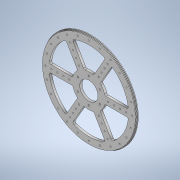
# Autodesk Inventor part: IndexerWheelV2
Saved by Autodesk Inventor 2020 (Build 240168000, 168)
## iProperties
Created: 2020-01-26
Part Number: IndexerWheelV2
Material: Generic
Document SubType Name: Modeling
Designer: srini
Density: 1 g/cm^3
Appearance: Default
Author: srini
Autodesk Inventor part; units mm, degrees
ref_plane "YZ Plane" through (0, 0, 0) normal (1, 0, 0) x (0, 1, 0)
ref_plane "XZ Plane" through (0, 0, 0) normal (0, 1, 0) x (-1, 0, 0)
ref_plane "XY Plane" through (0, 0, 0) normal (0, 0, 1) x (1, 0, 0)
sketch "Sketch1" plane through (0, 0, 0) normal (0, 0, 1) x (1, 0, 0)
  circle A0 centre (0, 0) radius 200.025
  circle A1 centre (0, 0) radius 38.4
  circle A2 centre (0, 53.975) radius 3.3734
  circle A3 centre (-46.7437, 26.9875) radius 3.3734
  circle A4 centre (-46.7437, -26.9875) radius 3.3734
  circle A5 centre (0, -53.975) radius 3.3734
  circle A6 centre (46.7437, -26.9875) radius 3.3734
  circle A7 centre (46.7437, 26.9875) radius 3.3734
  arc A8 (70.0141, 153.018) -> (-70.0141, 153.018) centre (0, 0) ccw
  line L0 (-70.0141, 153.018) -> (-20.2629, 66.8464)
  arc A9 (20.2629, 66.8464) -> (-20.2629, 66.8464) centre (0, 0) ccw
  line L1 (20.2629, 66.8464) -> (70.0141, 153.018)
  line L2 (0, 168.275) -> (0, 69.85) construction
  arc A10 (-97.5104, 137.143) -> (-167.5245, 15.875) centre (0, 0) ccw
  line L3 (-167.5245, 15.875) -> (-68.0221, 15.875)
  arc A11 (-47.7592, 50.9714) -> (-68.0221, 15.875) centre (0, 0) ccw
  line L4 (-47.7592, 50.9714) -> (-97.5104, 137.143)
  arc A12 (-167.5245, -15.875) -> (-97.5104, -137.143) centre (0, 0) ccw
  line L5 (-97.5104, -137.143) -> (-47.7592, -50.9714)
  arc A13 (-68.0221, -15.875) -> (-47.7592, -50.9714) centre (0, 0) ccw
  line L6 (-68.0221, -15.875) -> (-167.5245, -15.875)
  arc A14 (-70.0141, -153.018) -> (70.0141, -153.018) centre (0, 0) ccw
  line L7 (70.0141, -153.018) -> (20.2629, -66.8464)
  arc A15 (-20.2629, -66.8464) -> (20.2629, -66.8464) centre (0, 0) ccw
  line L8 (-20.2629, -66.8464) -> (-70.0141, -153.018)
  arc A16 (97.5104, -137.143) -> (167.5245, -15.875) centre (0, 0) ccw
  line L9 (167.5245, -15.875) -> (68.0221, -15.875)
  arc A17 (47.7592, -50.9714) -> (68.0221, -15.875) centre (0, 0) ccw
  line L10 (47.7592, -50.9714) -> (97.5104, -137.143)
  arc A18 (167.5245, 15.875) -> (97.5104, 137.143) centre (0, 0) ccw
  line L11 (97.5104, 137.143) -> (47.7592, 50.9714)
  arc A19 (68.0221, 15.875) -> (47.7592, 50.9714) centre (0, 0) ccw
  line L12 (68.0221, 15.875) -> (167.5245, 15.875)
  point P0 (-145.7304, 84.1375)
  point P1 (-60.4919, 34.925)
  point P2 (-145.7304, -84.1375)
  point P3 (-60.4919, -34.925)
  point P4 (0, -168.275)
  point P5 (0, -69.85)
  point P6 (145.7304, -84.1375)
  point P7 (60.4919, -34.925)
  point P8 (145.7304, 84.1375)
  point P9 (60.4919, 34.925)
  dimension "d0" = 400.05
  dimension "d1" = 76.8
  dimension "d2" = 53.975
  dimension "d3" = 6.7469
  dimension "d6" = 360
  dimension "d8" = 168.275
  dimension "d9" = 69.85
  dimension "d12" = 360
  dimension "d14" = 31.75
  constraints: 26 end point, 26 point on circle, 20 centre point, 2 coincident, 2 concentric, 1 parallel, 1 point on line, 1 vertical, 1 vertical alignment, 86 other
  measures "d0" diameter of A0
  measures "d1" diameter of A1
  measures "d2" distance of point (0, 0) A2.centre
  measures "d3" diameter of A2
  measures "d8" radius of A8
  measures "d9" radius of A9
  measures "d14" distance between parallel lines of L4 L0
extrude "Extrusion1" add sketch "Sketch1" along normal blind 9.525
fillet "Fillet1" radius 6.35 24 edges at (-167.5245, 15.875, 4.7625) (-70.0141, 153.018, 4.7625) (97.5104, 137.143, 4.7625) (167.5245, -15.875, 4.7625) (70.0141, -153.018, 4.7625) (-97.5104, -137.143, 4.7625) (-167.5245, -15.875, 4.7625) (-97.5104, 137.143, 4.7625) (70.0141, 153.018, 4.7625) (167.5245, 15.875, 4.7625) (97.5104, -137.143, 4.7625) (-70.0141, -153.018, 4.7625) (-68.0221, -15.875, 4.7625) (-47.7592, -50.9714, 4.7625) (-20.2629, -66.8464, 4.7625) (20.2629, -66.8464, 4.7625) (47.7592, -50.9714, 4.7625) (68.0221, -15.875, 4.7625) (68.0221, 15.875, 4.7625) (47.7592, 50.9714, 4.7625) (20.2629, 66.8464, 4.7625) (-20.2629, 66.8464, 4.7625) (-47.7592, 50.9714, 4.7625) (-68.0221, 15.875, 4.7625)
sketch "Sketch2" plane through (0, 0, 9.525) normal (0, 0, 1) x (1, 0, 0)
  circle A0 centre (0, 0) radius 198.4375
  circle A1 centre (0, 0) radius 200.025 projected
  dimension "d18" = 1.5875
  constraints: 1 centre point, 1 coincident
  measures "d18" radial gap between concentric circles of A0 A1
extrude "Extrusion2" cut sketch "Sketch2" against normal blind 6.35
sketch "Sketch3" plane through (0, 0, 9.525) normal (0, 0, 1) x (1, 0, 0)
  circle A0 centre (0, 0) radius 196.85
  circle A1 centre (0, 0) radius 198.4375 projected
  dimension "d21" = 1.5875
  constraints: 1 centre point, 1 coincident
  measures "d21" radial gap between concentric circles of A0 A1
extrude "Extrusion3" cut sketch "Sketch3" against normal blind 3.175
sketch "Sketch5" plane through (0, 0, 9.525) normal (0, 0, 1) x (1, 0, 0)
  circle A0 centre (-184.15, 0) radius 2.5781
  line L0 (-72.8868, 15.875) -> (-160.3925, 15.875) projected
  circle A1 centre (-158.75, 0) radius 2.5781
  circle A2 centre (-133.35, 0) radius 2.5781
  circle A3 centre (-107.95, 0) radius 2.5781
  circle A4 centre (-82.55, 0) radius 2.5781
  circle A5 centre (-79.375, -137.4815) radius 2.5781
  circle A6 centre (-66.675, -115.4845) radius 2.5781
  circle A7 centre (-53.975, -93.4874) radius 2.5781
  circle A8 centre (-41.275, -71.4904) radius 2.5781
  circle A9 centre (79.375, -137.4815) radius 2.5781
  circle A10 centre (66.675, -115.4845) radius 2.5781
  circle A11 centre (53.975, -93.4874) radius 2.5781
  circle A12 centre (41.275, -71.4904) radius 2.5781
  circle A13 centre (158.75, 0) radius 2.5781
  circle A14 centre (133.35, 0) radius 2.5781
  circle A15 centre (107.95, 0) radius 2.5781
  circle A16 centre (82.55, 0) radius 2.5781
  circle A17 centre (79.375, 137.4815) radius 2.5781
  circle A18 centre (66.675, 115.4845) radius 2.5781
  circle A19 centre (53.975, 93.4874) radius 2.5781
  circle A20 centre (41.275, 71.4904) radius 2.5781
  circle A21 centre (-79.375, 137.4815) radius 2.5781
  circle A22 centre (-66.675, 115.4845) radius 2.5781
  circle A23 centre (-53.975, 93.4874) radius 2.5781
  circle A24 centre (-41.275, 71.4904) radius 2.5781
  circle A25 centre (-177.8752, 47.6615) radius 2.5781
  circle A26 centre (-159.4786, 92.075) radius 2.5781
  circle A27 centre (-130.2137, 130.2137) radius 2.5781
  circle A28 centre (-92.075, 159.4786) radius 2.5781
  circle A29 centre (-47.6615, 177.8752) radius 2.5781
  circle A30 centre (0, 184.15) radius 2.5781
  circle A31 centre (47.6615, 177.8752) radius 2.5781
  circle A32 centre (92.075, 159.4786) radius 2.5781
  circle A33 centre (130.2137, 130.2137) radius 2.5781
  circle A34 centre (159.4786, 92.075) radius 2.5781
  circle A35 centre (177.8752, 47.6615) radius 2.5781
  circle A36 centre (184.15, 0) radius 2.5781
  circle A37 centre (177.8752, -47.6615) radius 2.5781
  circle A38 centre (159.4786, -92.075) radius 2.5781
  circle A39 centre (130.2137, -130.2137) radius 2.5781
  circle A40 centre (92.075, -159.4786) radius 2.5781
  circle A41 centre (47.6615, -177.8752) radius 2.5781
  circle A42 centre (0, -184.15) radius 2.5781
  circle A43 centre (-47.6615, -177.8752) radius 2.5781
  circle A44 centre (-92.075, -159.4786) radius 2.5781
  circle A45 centre (-130.2137, -130.2137) radius 2.5781
  circle A46 centre (-159.4786, -92.075) radius 2.5781
  circle A47 centre (-177.8752, -47.6615) radius 2.5781
  point P0 (0, 0)
  dimension "d24" = 5.1562
  dimension "d25" = 184.15
  dimension "d28" = 25.4
  dimension "d35" = 360
  dimension "d39" = 360
  constraints: 48 centre point, 1 horizontal, 1 horizontal alignment, 106 other
  measures "d24" diameter of A0
  measures "d25" distance of point (0, 0) A0.centre
  measures "d28" distance of A0.centre A1.centre
extrude "Extrusion4" cut sketch "Sketch5" against normal through all
equation "\"d2\" = 0.5 * InnerWheelDiameter + 0.5 * WebThick"
equation "\"d8\" = 0.5 * d0 - WebThick"
equation "\"d9\" = 0.5 * InnerWheelDiameter + WebThick"
equation "\"d14\" = WebThick"
equation "\"d19\" = 0.666667 * d15"
equation "\"d22\" = 0.333333 * d15"
equation "\"InnerWheelDiameter\" = 76.2"
equation "\"WebThick\" = 31.75"
equation "\"d15\" = 9.525"
body "Solid1"
